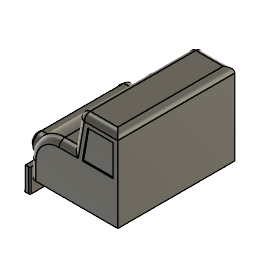
Truck Cabin (Autodesk Fusion 360 design; units mm, degrees)
part number: 2026-03-04-18-16-15-259
Autodesk Fusion 360 part; units mm, degrees
sketch "Sketch1" plane through (0, 0, 0) normal (0, 0, 1) x (1, 0, 0)
  line L0 (19.05, -25.4) -> (-19.05, -25.4)
  line L1 (-19.05, -25.4) -> (-19.05, 25.4)
  line L2 (-19.05, 25.4) -> (19.05, 25.4)
  line L3 (19.05, 25.4) -> (19.05, -25.4)
  line L4 (19.05, -25.4) -> (-19.05, 25.4) construction
  line L5 (-19.05, -25.4) -> (19.05, 25.4) construction
  dimension "d1" = 50.8
  dimension "d2" = 38.1
  constraint horizontal L0
  constraint perpendicular L0 L1
  constraint parallel L0 L2
  constraint parallel L1 L3
  constraint coincident L4 origin
  constraint coincident L5 origin
  measures "d1" distance of L0.end L1.end
  measures "d2" distance of L1.end L2.end
extrude "Extrude1" add sketch "Sketch1" along normal blind 20.32 makes body 1
sketch "Sketch2" plane through (0, 0, 20.32) normal (0, 0, 1) x (-1, 0, 0)
  line L0 (-19.05, -25.4) -> (19.05, -25.4)
  line L1 (19.05, -25.4) -> (19.05, 25.4)
  line L2 (19.05, 25.4) -> (-19.05, 25.4)
  line L3 (-19.05, 25.4) -> (-19.05, -25.4)
  line L4 (-19.05, 25.4) -> (3.81, 25.4)
  line L5 (3.81, 25.4) -> (3.81, -25.4)
  line L6 (3.81, -25.4) -> (-19.05, -25.4)
  line L7 (-19.05, -25.4) -> (-19.05, 25.4)
  dimension "d31" = 22.86
  constraint horizontal L4
  constraint vertical L5
  constraint horizontal L6
  constraint vertical L7
  constraint coincident L0 L5.end
  constraint coincident L2.end L3.start
  measures "d31" distance of L5.end L0.start
extrude "Extrude4" add sketch "Sketch2" along normal blind 15.24 contours L0 L2 L3 L4 L5 L6 L7 bodies 1
fillet "Fillet8" radius 12.7 1 edges at (-19.05, 0, 20.32) on bodies 1
draft "Draft1" angle -10 neutral plane through (0, 0, 0) pull (0, 0, -1) 1 faces at (-3.81, -8.4667, 30.48) on bodies 1
fillet "Fillet9" radius 2.54 12 edges at (-19.05, -25.4, 3.81) (-15.3303, -25.4, 16.6003) (-3.2885, -25.4, 20.32) (1.1166, -25.4, 27.94) (-3.2885, 25.4, 20.32) (-15.3303, 25.4, 16.6003) (-19.05, 25.4, 3.81) (1.1166, 25.4, 27.94) (2.4602, 0, 35.56) (10.7551, 25.4, 35.56) (10.7551, -25.4, 35.56) (19.05, 0, 35.56) on bodies 1
sketch "Sketch6" plane through (0, -25.4, 0) normal (0, -1, 0) x (1, 0, 0)
  line L0 (19.05, 33.02) -> (4.5915, 33.02)
  line L1 (4.5915, 33.02) -> (1.9043, 17.78)
  line L2 (1.9043, 17.78) -> (-6.35, 17.78)
  arc A0 (-6.35, 17.78) -> (-16.51, 7.62) centre (-6.35, 7.62) ccw
  line L3 (-16.51, 7.62) -> (-16.51, 0)
  line L4 (-16.51, 0) -> (19.05, 0)
  line L5 (19.05, 0) -> (19.05, 33.02)
  line L6 (6.0834, 31.242) -> (3.7097, 17.78)
  line L7 (3.7097, 17.78) -> (17.018, 17.78)
  line L8 (17.018, 17.78) -> (17.018, 31.242)
  line L9 (17.018, 31.242) -> (6.0834, 31.242)
  dimension "d59" = 2.032
  dimension "d60" = 1.778
  dimension "d61" = 1.778
  constraint horizontal L7
  constraint perpendicular L7 L8
  constraint parallel L0 L9
  constraint parallel L1 L6
  constraint collinear L2 L7
  measures "d59" distance of L5 L8
  measures "d60" distance of L0 L9
  measures "d61" distance of L1 L6
extrude "Extrude8" cut sketch "Sketch6" against normal blind 1.27 contours L6 L7 L8 L9 bodies 1
mirror "Mirror2" about plane through (0, 0, 0) normal (0, 1, 0) of "Extrude8"
sketch "Sketch3" plane through (-3.6951, 0, 0.6515) normal (-0.984808, 0, 0.173648) x (0, -1, 0)
  line L0 (-22.86, 33.3157) -> (-22.86, 19.9719)
  line L1 (-22.86, 19.9719) -> (22.86, 19.9719)
  line L2 (22.86, 19.9719) -> (22.86, 33.3157)
  line L3 (22.86, 33.3157) -> (-22.86, 33.3157)
  line L4 (-21.59, 31.7917) -> (21.59, 31.7917)
  line L5 (21.59, 31.7917) -> (21.59, 21.6317)
  line L6 (21.59, 21.6317) -> (-21.59, 21.6317)
  line L7 (-21.59, 21.6317) -> (-21.59, 31.7917)
  dimension "d40" = 43.18
  dimension "d41" = 10.16
  dimension "d42" = 1.524
  dimension "d43" = 1.27
  constraint horizontal L4
  constraint vertical L5
  constraint horizontal L6
  constraint vertical L7
  measures "d40" distance of L4.start L4.end
  measures "d41" distance of L4.start L6.end
  measures "d42" distance of L3 L4
  measures "d43" distance of L0 L7
extrude "Extrude5" cut sketch "Sketch3" against normal blind 1.27 contours L4 L5 L6 L7 bodies 1
sketch "Sketch4" plane through (-19.05, 0, 0) normal (-1, 0, 0) x (0, -1, 0)
  line L0 (-22.86, 7.62) -> (-22.86, 0)
  line L1 (-22.86, 0) -> (22.86, 0)
  line L2 (22.86, 0) -> (22.86, 7.62)
  line L3 (22.86, 7.62) -> (-22.86, 7.62)
  line L4 (-21.59, 12.7) -> (21.59, 12.7)
  line L5 (21.59, 12.7) -> (21.59, 5.08)
  line L6 (21.59, 5.08) -> (-21.59, 5.08)
  line L7 (-21.59, 5.08) -> (-21.59, 12.7)
  dimension "d46" = 1.27
  dimension "d47" = 1.27
  dimension "d48" = 7.62
  dimension "d49" = 5.08
  constraint horizontal L4
  constraint vertical L5
  constraint horizontal L6
  constraint vertical L7
  measures "d46" distance of L0 L7
  measures "d47" distance of L2 L5
  measures "d48" distance of L4 L6
  measures "d49" distance of L1 L6
extrude "Extrude6" add sketch "Sketch4" along normal blind 2.54 and the other way blind 1.27 separate body contours L3 L4 L5 L7 | L3 L5 L6 L7 makes body 2
fillet "Fillet10" radius 3.81 4 edges at (-19.685, -21.59, 12.7) (-19.685, -21.59, 5.08) (-19.685, 21.59, 12.7) (-19.685, 21.59, 5.08) on bodies 2
sketch "Sketch5" plane through (-21.59, 0, 0) normal (-1, 0, 0) x (0, -1, 0)
  arc A0 (-17.78, 12.7) -> (-17.78, 5.08) centre (-17.78, 8.89) ccw
  line L0 (-17.78, 5.08) -> (17.78, 5.08)
  arc A1 (17.78, 5.08) -> (17.78, 12.7) centre (17.78, 8.89) ccw
  line L1 (17.78, 12.7) -> (-17.78, 12.7)
  circle A2 centre (-17.78, 8.89) radius 2.8398
  circle A3 centre (17.78, 8.89) radius 2.8398
  constraint concentric A0 A2
  constraint concentric A1 A3
extrude "Extrude7" add sketch "Sketch5" along normal blind 1.27 separate body contours A2 | A3 makes body 3 at (-21.59, 17.1792, 9.489) makes body 4 at (-21.59, -17.9859, 9.7501)
sketch "Sketch7" plane through (-21.59, 0, 0) normal (-1, 0, 0) x (0, -1, 0)
  arc A0 (-17.78, 12.7) -> (-17.78, 5.08) centre (-17.78, 8.89) ccw
  line L0 (-17.78, 5.08) -> (17.78, 5.08)
  arc A1 (17.78, 5.08) -> (17.78, 12.7) centre (17.78, 8.89) ccw
  line L1 (17.78, 12.7) -> (-17.78, 12.7)
  line L2 (-16.51, 11.43) -> (16.51, 11.43)
  line L3 (-15.4694, 10.541) -> (15.4694, 10.541)
  line L4 (-15.4694, 7.239) -> (15.4694, 7.239)
  line L5 (-14.986, 8.382) -> (14.986, 8.382)
  line L6 (-14.986, 9.398) -> (14.986, 9.398)
  line L7 (-16.51, 6.35) -> (16.51, 6.35)
  circle A2 centre (17.78, 8.89) radius 2.8398
  circle A3 centre (-17.78, 8.89) radius 2.8398
  dimension "d66" = 5.08
  dimension "d68" = 2.032
  dimension "d69" = 2.032
  dimension "d70" = 0.889
  dimension "d71" = 0.889
  constraint parallel L1 L2
  constraint parallel L2 L3
  constraint parallel L3 L4
  constraint parallel L4 L5
  constraint parallel L0 L6
  constraint parallel L0 L7
  constraint coincident L2.end A2
  constraint coincident L3.end A2
  constraint coincident L6.end A2
  constraint coincident L5.end A2
  constraint coincident L4.end A2
  constraint coincident L7.end A2
  constraint coincident L2.start A3
  constraint coincident L3.start A3
  constraint coincident L6.start A3
  constraint coincident L5.start A3
  constraint coincident L4.start A3
  constraint coincident L7.start A3
  measures "d66" distance of L2 L7
  measures "d68" distance of L2 L6
  measures "d69" distance of L5 L7
  measures "d70" distance of L4 L7
  measures "d71" distance of L2 L3
extrude "Extrude9" cut sketch "Sketch7" against normal blind 1.27 contours L2 L3 A2 A3 | L4 L7 A2 A3 | L5 L6 A2 A3 bodies 4 3 2 1
sketch "Sketch8" plane through (0, 0, 0) normal (0, 0, -1) x (1, 0, 0)
  arc A0 (-19.05, -22.86) -> (-16.51, -25.4) centre (-16.51, -22.86) ccw
  line L0 (-16.51, -25.4) -> (19.05, -25.4)
  line L1 (19.05, -25.4) -> (19.05, 25.4)
  line L2 (19.05, 25.4) -> (-16.51, 25.4)
  arc A1 (-16.51, 25.4) -> (-19.05, 22.86) centre (-16.51, 22.86) ccw
  line L3 (-19.05, 22.86) -> (-19.05, -22.86)
  circle A2 centre (0, 0) radius 3.5
  dimension "d76" = 7
  constraint coincident A2.centre origin
  measures "d76" diameter of A2
extrude "Extrude10" cut sketch "Sketch8" against normal blind 2 contours A2 bodies 1
sketch "Sketch9" plane through (-19.05, 0, 0) normal (-1, 0, 0) x (0, -1, 0)
  line L0 (-22.86, 7.62) -> (-22.86, 0)
  line L1 (-22.86, 0) -> (22.86, 0)
  line L2 (22.86, 0) -> (22.86, 7.62)
  line L3 (22.86, 7.62) -> (-22.86, 7.62)
  line L4 (-25.4, 3.81) -> (25.4, 3.81)
  line L5 (25.4, 3.81) -> (25.4, -6.35)
  line L6 (25.4, -6.35) -> (-25.4, -6.35)
  line L7 (-25.4, -6.35) -> (-25.4, 3.81)
  line L8 (0, 1.75) -> (0, 22.5)
  dimension "d79" = 50.8
  dimension "d80" = 10.16
  dimension "d81" = 3.81
  constraint horizontal L4
  constraint vertical L5
  constraint horizontal L6
  constraint vertical L7
  constraint symmetric L5 L7 L8
  measures "d79" distance of L4.start L4.end
  measures "d80" distance of L4 L6
  measures "d81" distance of L1 L4
extrude "Extrude11" add sketch "Sketch9" along normal blind 2.54 separate body contours L0 L1 L2 L4 | L0 L1 L2 L4 L5 L6 L7 makes body 5
fillet "Fillet11" radius 0.508 2 edges at (-19.05, -25.4, -1.27) (-19.05, 25.4, -1.27) 1 faces at (-21.59, 0, -2.9633) on bodies 5
sketch "Sketch10" plane through (-2.4444, 0, 0.431) normal (-0.984808, 0, 0.173648) x (0, -1, 0)
  line L0 (-21.59, 21.6317) -> (21.59, 21.6317)
  line L1 (21.59, 21.6317) -> (21.59, 31.7917)
  line L2 (21.59, 31.7917) -> (-21.59, 31.7917)
  line L3 (-21.59, 31.7917) -> (-21.59, 21.6317)
extrude "Extrude12" add sketch "Sketch10" along normal blind 0.762 separate body makes body 6
sketch "Sketch11" plane through (0, -24.13, 0) normal (0, -1, 0) x (1, 0, 0)
  line L0 (17.018, 31.242) -> (6.0834, 31.242)
  line L1 (6.0834, 31.242) -> (3.7097, 17.78)
  line L2 (3.7097, 17.78) -> (17.018, 17.78)
  line L3 (17.018, 17.78) -> (17.018, 31.242)
extrude "Extrude13" add sketch "Sketch11" along normal blind 0.762 separate body makes body 7
sketch "Sketch12" plane through (0, 24.13, 0) normal (0, 1, 0) x (-1, 0, 0)
  line L0 (-6.0834, 31.242) -> (-17.018, 31.242)
  line L1 (-17.018, 31.242) -> (-17.018, 17.78)
  line L2 (-17.018, 17.78) -> (-3.7097, 17.78)
  line L3 (-3.7097, 17.78) -> (-6.0834, 31.242)
extrude "Extrude14" add sketch "Sketch12" along normal blind 0.762 separate body makes body 8
